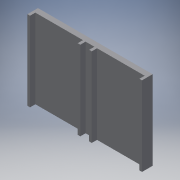
# Autodesk Inventor part: base_2
Saved by Autodesk Inventor 2019 (Build 230136000, 136)
## iProperties
Created: 2020-03-13
Part Number: base_2
Material: Generic
Document SubType Name: Modeling
Designer: Pulag
Density: 1 g/cm^3
Appearance: Default
Author: Pulag
Autodesk Inventor part; units mm, degrees
ref_plane "YZ Plane" through (0, 0, 0) normal (1, 0, 0) x (0, 1, 0)
ref_plane "XZ Plane" through (0, 0, 0) normal (0, 1, 0) x (-1, 0, 0)
ref_plane "XY Plane" through (0, 0, 0) normal (0, 0, 1) x (1, 0, 0)
sketch "Sketch1" plane through (0, 0, 0) normal (0, 0, 1) x (1, 0, 0)
  line L0 (0.75, -26.5) -> (0.75, 26.5) projected
  line L1 (0.75, 26.5) -> (-0.75, 26.5) projected
  line L2 (-0.75, 26.5) -> (-0.75, -26.5) projected
  line L3 (-0.75, -26.5) -> (0.75, -26.5) projected
  line L4 (27.75, 26.5) -> (27.75, -26.5) projected
  line L5 (27.75, -26.5) -> (29.25, -26.5) projected
  line L6 (29.25, -26.5) -> (29.25, 26.5) projected
  line L7 (29.25, 26.5) -> (27.75, 26.5) projected
  line L8 (35.75, -26.5) -> (35.75, 26.5) projected
  line L9 (35.75, 26.5) -> (34.25, 26.5) projected
  line L10 (34.25, 26.5) -> (34.25, -26.5) projected
  line L11 (34.25, -26.5) -> (35.75, -26.5) projected
  line L12 (64.25, -26.5) -> (64.25, 26.5) projected
  line L13 (62.75, 26.5) -> (62.75, -26.5) projected
  line L14 (62.75, -26.5) -> (64.25, -26.5) projected
  line L15 (64.25, -26.5) -> (64.25, 26.5) projected
  line L16 (64.25, 26.5) -> (62.75, 26.5) projected
  line L17 (64.25, -26.5) -> (-0.75, -26.5)
  line L18 (-0.75, -26.5) -> (-0.75, 18.5)
  line L19 (-0.75, 18.5) -> (64.25, 18.5)
  line L20 (64.25, 18.5) -> (64.25, -26.5)
  line L21 (62.75, 18.5) -> (62.75, -26.5)
  line L22 (35.75, 18.5) -> (35.75, -26.5)
  line L23 (34.25, 18.5) -> (34.25, -26.5)
  line L24 (29.25, 18.5) -> (29.25, -26.5)
  line L25 (27.75, -26.5) -> (27.75, 18.5)
  line L26 (0.75, 18.5) -> (0.75, -26.5)
  point P0 (0, 0)
  dimension "d0" = 45
  constraints: 20 end point, 13 point on line, 4 collinear, 2 parallel, 2 perpendicular, 1 horizontal
  measures "d0" distance of L17.end L18.end
extrude "Extrusion1" add sketch "Sketch1" along normal blind 3 contours L3 L2 L19 L0 | L0 L19 L4 L17 | L4 L19 L6 L5 | L6 L19 L10 L17 | L10 L19 L8 L11 | L8 L19 L13 L17 | L13 L19 L12 L14
sketch "Sketch2" plane through (0, 0, 3) normal (0, 0, 1) x (1, 0, 0)
  line L0 (0.75, -26.5) -> (0.75, 26.5)
  line L1 (0.75, 26.5) -> (-0.75, 26.5)
  line L2 (-0.75, 26.5) -> (-0.75, -26.5)
  line L3 (-0.75, -26.5) -> (0.75, -26.5)
  line L4 (27.75, 26.5) -> (27.75, -26.5)
  line L5 (27.75, -26.5) -> (29.25, -26.5)
  line L6 (29.25, -26.5) -> (29.25, 26.5)
  line L7 (29.25, 26.5) -> (27.75, 26.5)
  line L8 (35.75, -26.5) -> (35.75, 26.5)
  line L9 (35.75, 26.5) -> (34.25, 26.5)
  line L10 (34.25, 26.5) -> (34.25, -26.5)
  line L11 (34.25, -26.5) -> (35.75, -26.5)
  line L12 (64.25, -26.5) -> (64.25, 26.5)
  line L13 (62.75, 26.5) -> (62.75, -26.5)
  line L14 (62.75, -26.5) -> (64.25, -26.5)
  line L15 (64.25, -26.5) -> (64.25, 26.5)
  line L16 (64.25, 26.5) -> (62.75, 26.5)
  line L17 (64.25, -26.5) -> (-0.75, -26.5)
  line L18 (-0.75, -26.5) -> (-0.75, 18.5)
  line L19 (-0.75, 18.5) -> (64.25, 18.5)
  line L20 (64.25, 18.5) -> (64.25, -26.5)
  line L21 (62.75, 18.5) -> (62.75, -26.5)
  line L22 (35.75, 18.5) -> (35.75, -26.5)
  line L23 (34.25, 18.5) -> (34.25, -26.5)
  line L24 (29.25, 18.5) -> (29.25, -26.5)
  line L25 (27.75, -26.5) -> (27.75, 18.5)
  line L26 (0.75, 18.5) -> (0.75, -26.5)
  line L27 (0.75, -26.5) -> (0.75, 26.5)
  line L28 (0.75, 26.5) -> (-0.75, 26.5)
  line L29 (-0.75, 26.5) -> (-0.75, -26.5)
  line L30 (-0.75, -26.5) -> (0.75, -26.5)
  line L31 (27.75, 26.5) -> (27.75, -26.5)
  line L32 (27.75, -26.5) -> (29.25, -26.5)
  line L33 (29.25, -26.5) -> (29.25, 26.5)
  line L34 (29.25, 26.5) -> (27.75, 26.5)
  line L35 (35.75, -26.5) -> (35.75, 26.5)
  line L36 (35.75, 26.5) -> (34.25, 26.5)
  line L37 (34.25, 26.5) -> (34.25, -26.5)
  line L38 (34.25, -26.5) -> (35.75, -26.5)
  line L39 (64.25, -26.5) -> (64.25, 26.5)
  line L40 (62.75, 26.5) -> (62.75, -26.5)
  line L41 (62.75, -26.5) -> (64.25, -26.5)
  line L42 (64.25, -26.5) -> (64.25, 26.5)
  line L43 (64.25, 26.5) -> (62.75, 26.5)
  line L44 (64.25, -26.5) -> (-0.75, -26.5)
  line L45 (-0.75, -26.5) -> (-0.75, 18.5)
  line L46 (-0.75, 18.5) -> (64.25, 18.5)
  line L47 (64.25, 18.5) -> (64.25, -26.5)
  line L48 (62.75, 18.5) -> (62.75, -26.5)
  line L49 (35.75, 18.5) -> (35.75, -26.5)
  line L50 (34.25, 18.5) -> (34.25, -26.5)
  line L51 (29.25, 18.5) -> (29.25, -26.5)
  line L52 (27.75, -26.5) -> (27.75, 18.5)
  line L53 (0.75, 18.5) -> (0.75, -26.5)
  point P0 (0, 0)
  point P1 (0, 0)
  point P2 (0, 0)
  dimension "d3" = 45
  dimension "d4" = 45
  constraints: 108 end point, 26 point on line, 8 collinear, 4 parallel, 4 perpendicular, 2 horizontal
  measures "d3" distance of L17.end L18.end
  measures "d4" distance of L44.end L45.end
extrude "Extrusion2" add sketch "Sketch2" along normal blind 3 contours L3 L2 L19 L0 | L4 L19 L6 L5 | L10 L19 L8 L11 | L13 L19 L12 L14
body "Solid1"
